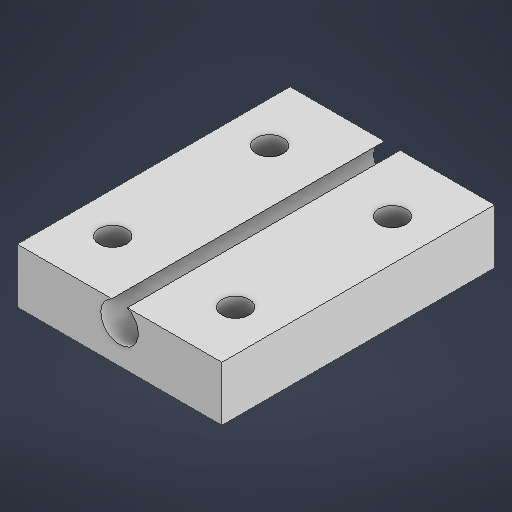
# Autodesk Inventor part: Differential_drive_wheel
Saved by Autodesk Inventor 2026 (Build 300175000, 175)
## iProperties
Created: 2025-07-10
Part Number: Differential_drive_wheel
Material: Generic
Document SubType Name: Modeling
Designer: user
Density: 1 g/cm^3
Appearance: Default
Author: user
Autodesk Inventor part; units mm, degrees
ref_plane "YZ Plane" through (0, 0, 0) normal (1, 0, 0) x (0, 1, 0)
ref_plane "XZ Plane" through (0, 0, 0) normal (0, 1, 0) x (-1, 0, 0)
sketch "Sketch1" plane through (0, 0, 0) normal (0, 0, 1) x (1, 0, 0)
  line L0 (-15, -4) -> (15, -4)
  line L1 (15, -4) -> (15, 4)
  line L2 (15, 4) -> (-15, 4)
  line L3 (-15, 4) -> (-15, -4)
  line L4 (-15, -4) -> (15, 4) construction
  line L5 (15, -4) -> (-15, 4) construction
  point P0 (0, 0)
  dimension "d2" = 30
  dimension "d3" = 8
  constraints: 12 end point, 2 midpoint, 2 parallel, 1 horizontal, 1 perpendicular
  measures "d2" distance of L2.end L1.end
  measures "d3" distance of L1.end L0.end
extrude "Extrusion1" add sketch "Sketch1" against normal blind 40
sketch "Sketch2" plane through (0, 0, 0) normal (0, 0, 1) x (1, 0, 0)
  circle A0 centre (0, 1.5) radius 2.75
  line L0 (-15, -4) -> (15, -4) projected
  point P0 (0, 0)
  point P1 (-9, -4)
  point P2 (9, -4)
  dimension "d7" = 5.5
  dimension "d8" = 5.5
  constraints: 1 centre point
  measures "d7" diameter of A0
  measures "d8" distance from line of L0 A0.centre
extrude "Extrusion2" cut sketch "Sketch2" against normal blind 40
sketch "Sketch3" plane through (15, 4, 0) normal (0, 1, 0) x (1, 0, 0)
  circle A0 centre (-6, 8) radius 2
  line L0 (0, 0) -> (0, 40) projected
  line L1 (0, 0) -> (-13.8544, 0) projected
  point P0 (-15, 0)
  dimension "d11" = 4
  dimension "d12" = 6
  dimension "d13" = 8
  constraints: 1 centre point
  measures "d11" diameter of A0
  measures "d12" distance from line of L0 A0.centre
  measures "d13" distance from line of L1 A0.centre
extrude "Extrusion3" cut sketch "Sketch3" against normal blind 40
pattern_linear "Rectangular Pattern1" count 2 spacing 23 along (0, 0, -1) of "Extrusion3"
ref_plane "Work Plane1" through (0, -4, 0) normal (1, 0, 0) x (0, 0, -1)
mirror "Mirror1" about plane through (0, -4, 0) normal (1, 0, 0) of "Extrusion3", "Rectangular Pattern1"
body "Solid1"
